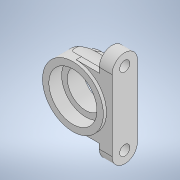
# Autodesk Inventor part: Крепление дифференциала
Saved by Autodesk Inventor 2020 (Build 240168000, 168)
## iProperties
Created: 2021-05-24
Part Number: Крепление дифференциала
Material: Типовые
Document SubType Name: Modeling
Designer: Антон
Density: 1 g/cm^3
Appearance: По умолчанию
Author: Антон
Autodesk Inventor part; units mm, degrees
ref_plane "YZ Plane" through (0, 0, 0) normal (1, 0, 0) x (0, 1, 0)
ref_plane "XZ Plane" through (0, 0, 0) normal (0, 1, 0) x (-1, 0, 0)
sketch "Эскиз1" plane through (0, 0, 0) normal (0, 0, 1) x (1, 0, 0)
  circle A0 centre (0, 0) radius 5.75
  circle A1 centre (0, 0) radius 9.55
  dimension "d0" = 11.5
  dimension "d1" = 19.1
  constraints: 2 centre point, 2 coincident
  measures "d0" diameter of A0
  measures "d1" diameter of A1
extrude "Выдавливание1" add sketch "Эскиз1" along normal blind 9
sketch "Эскиз2" plane through (0, 0, 9) normal (0, 0, 1) x (1, 0, 0)
  circle A0 centre (0, 0) radius 7.55
  dimension "d4" = 15.1
  constraints: 1 centre point, 1 coincident
  measures "d4" diameter of A0
extrude "Выдавливание2" cut sketch "Эскиз2" against normal blind 4
chamfer "Фаска1" distance 3 distance2 1.8 1 edges at (-9.55, 0, 0) measured on face at (9.519, -0.7685, 6)
sketch "Эскиз3" plane through (0, 0, 0) normal (0, 0, -1) x (-1, 0, 0)
  circle A0 centre (0, 0) radius 5.75 projected
  circle A1 centre (0, 0) radius 7.75 projected
  circle A2 centre (0, 0) radius 9.55 projected
  line L0 (0, 9.55) -> (-11.3, 9.55)
  line L1 (-11.3, 9.55) -> (-11.3, -9.55)
  line L2 (-11.3, -9.55) -> (0, -9.55)
  line L3 (0, -9.55) -> (0, 9.55)
  point P0 (0, -7.75)
  point P1 (0, 7.75)
  dimension "d10" = 11.3
  constraints: 8 end point, 2 horizontal, 2 parallel, 1 midpoint, 1 perpendicular, 1 vertical alignment, 1 other
  measures "d10" distance between parallel lines of L3 L1
extrude "Выдавливание3" add sketch "Эскиз3" against normal blind 8 contours A1 L3 A2 | A2 L2 L1 L0 picked at (-0.7618, -8.8575)
sketch "Эскиз4" plane through (0, 7.75, 0) normal (-1, 0, 0) x (0, 0, 1)
  line L0 (3, 1.8) -> (0, 0) projected
  line L1 (0, 1.8) -> (3, 1.8) projected
  line L2 (0, 0) -> (0, 1.8) projected
  line L3 (0, -17.3) -> (3, -17.3) projected
  line L4 (0, -15.5) -> (3, -17.3) projected
  line L5 (0, -17.3) -> (0, -15.5) projected
  line L6 (0, -17.3) -> (3, -17.3) projected
  point P0 (0, -7.75)
extrude "Выдавливание4" cut sketch "Эскиз4" against normal through all
sketch "Эскиз5" plane through (11.3, -9.55, 8) normal (1, 0, 0) x (0, 0, -1)
  line L0 (0, 19.1) -> (0, 0) projected
  line L1 (0, 19.1) -> (8, 19.1)
  line L2 (8, 19.1) -> (8, 24.7)
  line L3 (8, 24.7) -> (0, 24.7)
  line L4 (0, 24.7) -> (0, 19.1)
  line L5 (8, 19.1) -> (5, 19.1)
  line L6 (5, 19.1) -> (5, 16.7)
  line L7 (5, 16.7) -> (8, 16.7)
  line L8 (8, 16.7) -> (8, 19.1)
  line L9 (5, 0) -> (5, 19.1) projected
  point P0 (8, 9.55)
  dimension "d15" = 8
  dimension "d16" = 5.6
  dimension "d26" = 8
  constraints: 16 end point, 4 parallel, 2 horizontal, 2 perpendicular, 1 collinear
  measures "d15" distance of L3.end L2.end
  measures "d16" distance of L2.end L1.end
  measures "d26" distance between parallel lines of L3 L7
extrude "Выдавливание5" add sketch "Эскиз5" against normal blind 4
sketch "Эскиз6" plane through (7.3, -9.55, 8) normal (-1, 0, 0) x (0, 0, 1)
  line L0 (-5, 19.1) -> (-8, 17.3) projected
  line L1 (0, 19.1) -> (-5, 19.1) projected
  line L2 (0, 19.1) -> (0, 24.7) projected
  line L3 (0, 24.7) -> (-8, 24.7) projected
  line L4 (-8, 24.7) -> (-8, 17.3) projected
  line L5 (-8, 24.7) -> (-8, 17.3) projected
  line L6 (-8, 21) -> (0, 21)
  line L7 (0, 19.1) -> (0, 24.7) projected
  point P0 (-8, 9.55)
  point P1 (-4, 21)
  constraints: 2 end point, 2 midpoint, 1 perpendicular, 1 point on line
hole "Отверстие1" at (7.3, 11.45, 4) direction (1, 0, 0) diameter 3.2 end through all countersink diameter 6 countersink angle 90
sketch "Эскиз8" plane through (7.3, -9.55, 8) normal (-1, 0, 0) x (0, 0, 1)
  arc A0 (-1.6784, 19.1) -> (-5.8148, 18.6111) centre (-4, 21) ccw projected
  circle A1 centre (-4, 21) radius 1.6 projected
  arc A2 (-1.6784, 19.1) -> (-5.8148, 18.6111) centre (-4, 21) ccw projected
  arc A3 (-5.8148, 18.6111) -> (-1.6784, 19.1) centre (-4, 21) ccw projected
  circle A4 centre (-4, 21) radius 1.6 projected
  point P0 (-8, 9.55)
  point P1 (-5.8148, 18.6111)
  point P2 (-1.6784, 19.1)
extrude "Выдавливание6" cut sketch "Эскиз8" along normal through all contours A3 A0 | A1
fillet "Сопряжение1" radius 4 2 edges at (9.3, 15.15, 0) (9.3, 15.15, 8)
ref_plane "РабПлоскость1" through (0, 0, 8) normal (0, 1, 0) x (1, 0, 0)
mirror "Зеркальное отражение1" about plane through (0, 0, 8) normal (0, 1, 0) of "Сопряжение1", "Отверстие1", "Выдавливание6", "Выдавливание5"
